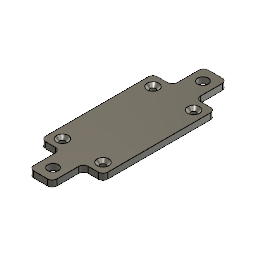
Hoverboard Final v3 (Autodesk Fusion 360 archive; units mm, degrees)
design "RPI PSU Bracket"
Autodesk Fusion 360 part; units mm, degrees
sketch "Sketch1" plane through (0, 0, 0) normal (0, 1, 0) x (1, 0, 0)
  line L0 (13, 29) -> (-13, 29) construction
  line L1 (-13, 29) -> (-13, -29) construction
  line L2 (-13, -29) -> (13, -29) construction
  line L3 (13, -29) -> (13, 29) construction
  line L4 (13, 29) -> (-13, -29) construction
  line L5 (-13, 29) -> (13, -29) construction
  line L6 (0, 0) -> (0, 16.0365) construction
  line L7 (0, 0) -> (-11.1519, 0) construction
  line L8 (20, 36) -> (-20, 36)
  line L9 (-20, 36) -> (-20, -36)
  line L10 (-20, -36) -> (20, -36)
  line L11 (20, -36) -> (20, 36)
  line L12 (20, 36) -> (-20, -36) construction
  line L13 (-20, 36) -> (20, -36) construction
  circle A0 centre (13, 29) radius 1.75
  circle A1 centre (-13, 29) radius 1.75
  circle A2 centre (13, -29) radius 1.75
  circle A3 centre (-13, -29) radius 1.75
  line L14 (7.5, 36) -> (-7.5, 36)
  line L15 (-7.5, 36) -> (-7.5, 56)
  line L16 (-7.5, 56) -> (7.5, 56)
  line L17 (7.5, 56) -> (7.5, 36)
  line L18 (7.5, 36) -> (-7.5, 56) construction
  line L19 (-7.5, 36) -> (7.5, 56) construction
  circle A4 centre (0, 48) radius 3.4
  line L20 (7.5, -56) -> (7.5, -36)
  line L21 (-7.5, -56) -> (7.5, -56)
  line L22 (-7.5, -36) -> (-7.5, -56)
  circle A5 centre (0, -48) radius 3.4
  line L23 (7.5, -36) -> (-7.5, -36)
  point P0 (0, 46)
  dimension "d1" = 3.5
  dimension "d2" = 58
  dimension "d3" = 26
  dimension "d4" = 7
  dimension "d5" = 7
  dimension "d6" = 15
  dimension "d7" = 20
  dimension "d8" = 6.8
  dimension "d9" = 12
  constraint perpendicular L0 L1
  constraint parallel L0 L2
  constraint parallel L1 L3
  constraint horizontal L0
  constraint coincident L4 L6.start
  constraint coincident L5 L6.start
  constraint coincident L6.start L7.start
  constraint vertical L6
  constraint perpendicular L1 L7
  constraint perpendicular L8 L9
  constraint parallel L8 L10
  constraint parallel L9 L11
  constraint horizontal L8
  constraint coincident L12 L6.start
  constraint coincident L13 L6.start
  constraint coincident L0.start L3.end
  constraint symmetric L6 A0 A1
  constraint symmetric L7 A0 A2
  constraint symmetric L7 A1 A3
  constraint perpendicular L14 L15
  constraint parallel L14 L16
  constraint parallel L15 L17
  constraint horizontal L14
  constraint coincident L18 P0
  constraint coincident L19 P0
  constraint coincident L6 P0
  constraint coincident L8 L14.start
  constraint coincident L6 A4.centre
  constraint symmetric L7 L14.start L20.end
  constraint symmetric L7 L14.end L22.start
  constraint symmetric L7 L15.end L21.start
  constraint symmetric L7 L16.end L20.start
  constraint symmetric L7 A4 A5
  measures "d1" diameter of A0
  measures "d2" distance of L0.start L2.end
  measures "d3" distance of L0.start L0.end
  measures "d4" distance of L0 L8
  measures "d5" distance of L3 L11
  measures "d6" distance of L15.end L16.end
  measures "d7" distance of L14.start L16.end
  measures "d8" diameter of A4
  measures "d9" distance of L8 A4.centre
extrude "Extrude1" add sketch "Sketch1" along normal blind 4
fillet "Fillet1" radius 3 12 edges at (7.5, 2, 36) (20, 2, 36) (7.5, 2, 56) (-7.5, 2, 56) (-20, 2, 36) (-7.5, 2, 36) (20, 2, -36) (7.5, 2, -36) (7.5, 2, -56) (-7.5, 2, -56) (-20, 2, -36) (-7.5, 2, -36)
chamfer "Chamfer1" distance 2 angle 45 4 edges at (-14.6316, 4, -29.6328) (11.3684, 4, -29.6328) (11.3684, 4, 28.3672) (-14.6316, 4, 28.3672)

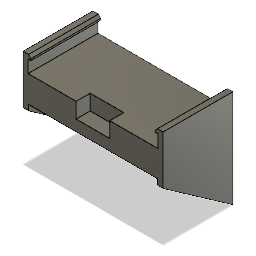
design "Sonar Bracket"
Autodesk Fusion 360 part; units mm, degrees
sketch "Sketch1" plane through (0, 0, 0) normal (0, 1, 0) x (1, 0, 0)
  line L0 (25, -12.5) -> (-25, -12.5)
  line L1 (-25, -12.5) -> (-25, 12.5)
  line L2 (-25, 12.5) -> (25, 12.5)
  line L3 (25, 12.5) -> (25, -12.5)
  line L4 (25, -12.5) -> (-25, 12.5) construction
  line L5 (-25, -12.5) -> (25, 12.5) construction
  dimension "d1" = 25
  dimension "d2" = 50
  constraint perpendicular L0 L1
  constraint parallel L0 L2
  constraint parallel L1 L3
  constraint horizontal L0
  constraint coincident L4 origin
  constraint coincident L5 origin
  measures "d1" distance of L0.end L1.end
  measures "d2" distance of L1.end L2.end
extrude "Extrude1" add sketch "Sketch1" along normal blind 35
sketch "Sketch2" plane through (0, 0, 12.5) normal (0, 0, 1) x (1, 0, 0)
  line L0 (-25, 0) -> (25, 0)
  line L1 (25, 0) -> (25, 35)
  line L2 (25, 35) -> (-25, 35)
  line L3 (-25, 35) -> (-25, 0)
  line L4 (0, 0) -> (0, 11) construction
  line L5 (23, 35) -> (22.15, 34.1)
  line L6 (22.15, 34.1) -> (22.15, 33.5)
  line L7 (22.15, 33.5) -> (23.15, 33.5)
  line L8 (23.15, 33.5) -> (23.15, 29)
  line L9 (23.15, 29) -> (0, 29)
  line L10 (23, 35) -> (0, 35)
  line L11 (-25, 35) -> (25, 35)
  line L12 (-23.15, 33.5) -> (-23.15, 29)
  line L13 (-25, 0) -> (-25, 35)
  line L14 (-23, 35) -> (0, 35)
  line L15 (-22.15, 33.5) -> (-23.15, 33.5)
  line L16 (-22.15, 34.1) -> (-22.15, 33.5)
  line L17 (-23.15, 29) -> (0, 29)
  line L18 (-23, 35) -> (-22.15, 34.1)
  dimension "d5" = 46.3
  dimension "d6" = 1
  dimension "d7" = 1.5
  dimension "d8" = 0.6
  dimension "d9" = 2
  dimension "d10" = 4.5
  constraint coincident L4.start origin
  constraint perpendicular L0 L4
  constraint coincident L2 L5.start
  constraint perpendicular L2 L6
  constraint perpendicular L6 L7
  constraint perpendicular L7 L8
  constraint perpendicular L6 L9
  constraint midpoint L2 L10.end
  constraint symmetric L0.end L4 L0.start
  constraint symmetric L1.end L4 L2.end
  constraint symmetric L2.end L4 L1.end
  constraint symmetric L4 L5.start L14.start
  constraint symmetric L4 L5.end L16.start
  constraint symmetric L4 L6.end L15.start
  constraint symmetric L4 L7.end L12.start
  constraint symmetric L4 L8.end L12.end
  constraint symmetric L4 L9.end L17.end
  constraint symmetric L4 L10.end L14.end
  measures "d5" distance of L8 L12
  measures "d6" distance of L6.end L7.end
  measures "d7" distance of L7.end L10
  measures "d8" distance of L5.end L6.end
  measures "d9" distance of L5.start L1.end
  measures "d10" distance of L7.end L8.end
extrude "Extrude2" cut sketch "Sketch2" against normal through all contours L2 L5 L6 L7 L8 L9 L10 L11 L12 L14 L15 L16 L17 L18
sketch "Sketch3" plane through (0, 0, 12.5) normal (0, 0, 1) x (1, 0, 0)
  line L0 (23, 35) -> (22.15, 34.1)
  line L1 (22.15, 34.1) -> (22.15, 33.5)
  line L2 (22.15, 33.5) -> (23.15, 33.5)
  line L3 (23.15, 33.5) -> (23.15, 29)
  line L4 (23.15, 29) -> (-23.15, 29)
  line L5 (-23.15, 29) -> (-23.15, 33.5)
  line L6 (-23.15, 33.5) -> (-22.15, 33.5)
  line L7 (-22.15, 33.5) -> (-22.15, 34.1)
  line L8 (-22.15, 34.1) -> (-23, 35)
  line L9 (-23, 35) -> (-25, 35)
  line L10 (-25, 35) -> (-25, 0)
  line L11 (-25, 0) -> (25, 0)
  line L12 (25, 0) -> (25, 35)
  line L13 (25, 35) -> (23, 35)
  line L14 (6, 23.5) -> (-6, 23.5)
  line L15 (-6, 23.5) -> (-6, 34.5)
  line L16 (-6, 34.5) -> (6, 34.5)
  line L17 (6, 34.5) -> (6, 23.5)
  line L18 (6, 23.5) -> (-6, 34.5) construction
  line L19 (-6, 23.5) -> (6, 34.5) construction
  point P0 (0, 29)
  dimension "d12" = 12
  dimension "d13" = 11
  constraint perpendicular L14 L15
  constraint parallel L14 L16
  constraint parallel L15 L17
  constraint horizontal L14
  constraint coincident L18 P0
  constraint coincident L19 P0
  constraint midpoint L4 P0
  measures "d12" distance of L14.start L14.end
  measures "d13" distance of L14.start L16.end
extrude "Extrude3" cut sketch "Sketch3" against normal blind 5 contours L4 L14 L15 L17
sketch "Sketch4" plane through (25, 0, 0) normal (1, 0, 0) x (0, 0, -1)
  line L0 (-12.5, 0) -> (12.5, 0)
  line L1 (12.5, 0) -> (12.5, 35)
  line L2 (12.5, 35) -> (-12.5, 35)
  line L3 (-12.5, 35) -> (-12.5, 0)
  line L4 (-12.5, 17.5) -> (12.5, 0)
  line L5 (12.5, 0) -> (-12.5, 0)
  line L6 (-12.5, 0) -> (-12.5, 17.5)
  constraint midpoint L3 L4.start
  constraint coincident L0.end L1.start
  constraint coincident L0.start L3.end
extrude "Extrude4" cut sketch "Sketch4" against normal through all contours L0 L3 L4 L5 L6
sketch "Sketch5" plane through (0, 0, 12.5) normal (0, 0, 1) x (1, 0, 0)
  line L0 (-25, 17.5) -> (25, 17.5)
  line L1 (25, 17.5) -> (25, 35)
  line L2 (25, 35) -> (23, 35)
  line L3 (23, 35) -> (22.15, 34.1)
  line L4 (22.15, 34.1) -> (22.15, 33.5)
  line L5 (22.15, 33.5) -> (23.15, 33.5)
  line L6 (23.15, 33.5) -> (23.15, 29)
  line L7 (23.15, 29) -> (6, 29)
  line L8 (6, 29) -> (6, 23.5)
  line L9 (6, 23.5) -> (-6, 23.5)
  line L10 (-6, 23.5) -> (-6, 29)
  line L11 (-6, 29) -> (-23.15, 29)
  line L12 (-23.15, 29) -> (-23.15, 33.5)
  line L13 (-23.15, 33.5) -> (-22.15, 33.5)
  line L14 (-22.15, 33.5) -> (-22.15, 34.1)
  line L15 (-22.15, 34.1) -> (-23, 35)
  line L16 (-23, 35) -> (-25, 35)
  line L17 (-25, 35) -> (-25, 17.5)
  line L18 (23, 19.5) -> (-23, 19.5)
  line L19 (-23, 19.5) -> (-23, 0)
  line L20 (-23, 0) -> (23, 0)
  line L21 (23, 0) -> (23, 19.5)
  line L22 (23, 19.5) -> (-23, 0) construction
  line L23 (-23, 19.5) -> (23, 0) construction
  line L24 (-25, 0) -> (25, 0)
  line L25 (25, 17.5) -> (25, 0)
  line L26 (-25, 0) -> (-25, 17.5)
  point P0 (0, 9.75)
  dimension "d17" = 2
  dimension "d18" = 2
  dimension "d19" = 2
  constraint perpendicular L18 L19
  constraint parallel L18 L20
  constraint parallel L19 L21
  constraint horizontal L18
  constraint coincident L22 P0
  constraint coincident L23 P0
  constraint collinear L20 L24
  measures "d17" distance of L0 L18
  measures "d18" distance of L21 L25
  measures "d19" distance of L19 L26
extrude "Extrude5" cut sketch "Sketch5" against normal blind 21 contours L0 L18 L19 L21 | L0 L19 L20 L21 L24
sketch "Sketch6" plane through (0, 0, -8.5) normal (0, 0, 1) x (1, 0, 0)
  line L0 (-23, 2.8) -> (23, 2.8)
  line L1 (23, 2.8) -> (23, 19.5)
  line L2 (23, 19.5) -> (-23, 19.5)
  line L3 (-23, 19.5) -> (-23, 2.8)
  circle A0 centre (0, 9.5) radius 3.25
  line L4 (0, 0) -> (0, 14) construction
  dimension "d22" = 6.5
  dimension "d23" = 9.5
  constraint coincident L4.start origin
  constraint vertical L4
  constraint coincident A0.centre L4
  measures "d22" diameter of A0
  measures "d23" distance of L4.start A0.centre
extrude "Extrude6" cut sketch "Sketch6" against normal through all contours A0

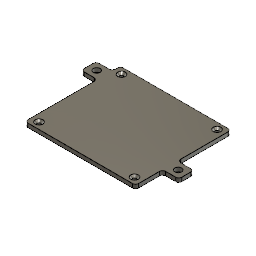
design "Power PCB Bracket"
Autodesk Fusion 360 part; units mm, degrees
sketch "Sketch1" plane through (0, 0, 0) normal (0, 1, 0) x (1, 0, 0)
  line L0 (47.35, 40.9) -> (-47.35, 40.9) construction
  line L1 (-47.35, 40.9) -> (-47.35, -40.9) construction
  line L2 (-47.35, -40.9) -> (47.35, -40.9) construction
  line L3 (47.35, -40.9) -> (47.35, 40.9) construction
  line L4 (47.35, 40.9) -> (-47.35, -40.9) construction
  line L5 (-47.35, 40.9) -> (47.35, -40.9) construction
  line L6 (54.9177, 47.4368) -> (-54.9177, 47.4368)
  line L7 (-54.9177, 47.4368) -> (-54.9177, -47.4368)
  line L8 (-54.9177, -47.4368) -> (54.9177, -47.4368)
  line L9 (54.9177, -47.4368) -> (54.9177, 47.4368)
  line L10 (54.9177, 47.4368) -> (-54.9177, -47.4368) construction
  line L11 (-54.9177, 47.4368) -> (54.9177, -47.4368) construction
  circle A0 centre (47.35, 40.9) radius 1.75
  line L12 (0, 0) -> (0, 35) construction
  line L13 (0, 0) -> (-41.0628, 0) construction
  circle A1 centre (-47.35, 40.9) radius 1.75
  circle A2 centre (47.35, -40.9) radius 1.75
  circle A3 centre (-47.35, -40.9) radius 1.75
  line L14 (-54.9177, 39.4) -> (-70.9177, 39.4)
  line L15 (-70.9177, 39.4) -> (-70.9177, 24.4)
  line L16 (-70.9177, 24.4) -> (-54.9177, 24.4)
  line L17 (-54.9177, 24.4) -> (-54.9177, 39.4)
  line L18 (54.9177, -5.6) -> (70.9177, -5.6)
  line L19 (70.9177, -5.6) -> (70.9177, -20.6)
  line L20 (70.9177, -20.6) -> (54.9177, -20.6)
  line L21 (54.9177, -20.6) -> (54.9177, -5.6)
  line L22 (81.8257, 31.9) -> (62.2169, 31.9) construction
  line L23 (80.3912, -13.1) -> (59.348, -13.1) construction
  circle A4 centre (-62.9177, 31.9) radius 3.4
  circle A5 centre (62.9177, -13.1) radius 3.4
  dimension "d1" = 3.5
  dimension "d2" = 81.8
  dimension "d3" = 94.7
  dimension "d4" = 10
  dimension "d5" = 16
  dimension "d6" = 15
  dimension "d7" = 15
  dimension "d9" = 16
  dimension "d10" = 45
  dimension "d11" = 9
  dimension "d12" = 6.8
  dimension "d13" = 6.8
  dimension "d14" = 8
  dimension "d15" = 8
  constraint perpendicular L0 L1
  constraint parallel L0 L2
  constraint parallel L1 L3
  constraint horizontal L0
  constraint coincident L4 L12.start
  constraint coincident L5 L12.start
  constraint coincident L12.start L13.start
  constraint perpendicular L6 L7
  constraint parallel L6 L8
  constraint parallel L7 L9
  constraint horizontal L6
  constraint coincident L10 L12.start
  constraint coincident L11 L12.start
  constraint collinear L4 L10
  constraint coincident L0.start L3.end
  constraint vertical L12
  constraint horizontal L13
  constraint symmetric A0 L12 A1
  constraint symmetric A0 L13 A2
  constraint symmetric L13 A1 A3
  constraint horizontal L14
  constraint vertical L15
  constraint horizontal L16
  constraint vertical L17
  constraint coincident L7 L14.start
  constraint horizontal L18
  constraint vertical L19
  constraint horizontal L20
  constraint vertical L21
  constraint coincident L9 L18.start
  constraint perpendicular L12 L22
  constraint symmetric L14 L16 L22
  constraint symmetric L18 L20 L23
  constraint coincident L23 A5.centre
  constraint coincident L22 A4.centre
  measures "d1" diameter of A0
  measures "d2" distance of L0.start L2.end
  measures "d3" distance of L0.start L0.end
  measures "d4" distance of L6.start L0.start
  measures "d5" distance of L14.start L14.end
  measures "d6" distance of L14.end L15.end
  measures "d7" distance of L18.end L19.end
  measures "d9" distance of L18.start L18.end
  measures "d10" distance of L22 L23
  measures "d11" distance of L0.end L22
  measures "d12" diameter of A5
  measures "d13" diameter of A4
  measures "d14" distance of L7 A4.centre
  measures "d15" distance of L21 A5.centre
extrude "Extrude1" add sketch "Sketch1" along normal blind 4
fillet "Fillet1" radius 3 12 edges at (-70.9177, 2, -24.4) (-70.9177, 2, -39.4) (-54.9177, 2, -39.4) (-54.9177, 2, -47.4368) (-54.9177, 2, 47.4368) (-54.9177, 2, -24.4) (54.9177, 2, 47.4368) (54.9177, 2, 20.6) (70.9177, 2, 20.6) (70.9177, 2, 5.6) (54.9177, 2, 5.6) (54.9177, 2, -47.4368)
chamfer "Chamfer1" distance 2 angle 45 4 edges at (45.7184, 4, 40.2672) (-48.9816, 4, 40.2672) (-48.9816, 4, -41.5328) (45.7184, 4, -41.5328)

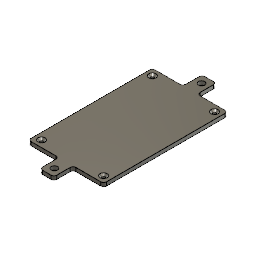
design "PSU Bracket"
Autodesk Fusion 360 part; units mm, degrees
sketch "Sketch1" plane through (0, 0, 0) normal (0, 1, 0) x (1, 0, 0)
  line L0 (32.5, 58) -> (-32.5, 58) construction
  line L1 (-32.5, 58) -> (-32.5, -58) construction
  line L2 (-32.5, -58) -> (32.5, -58) construction
  line L3 (32.5, -58) -> (32.5, 58) construction
  line L4 (32.5, 58) -> (-32.5, -58) construction
  line L5 (-32.5, 58) -> (32.5, -58) construction
  circle A0 centre (32.5, 58) radius 1.75
  line L6 (0, 0) -> (0, 14) construction
  line L7 (0, 0) -> (-15, 0) construction
  circle A1 centre (-32.5, 58) radius 1.75
  circle A2 centre (32.5, -58) radius 1.75
  circle A3 centre (-32.5, -58) radius 1.75
  line L8 (39.5, 65) -> (-39.5, 65)
  line L9 (-39.5, 65) -> (-39.5, -65)
  line L10 (-39.5, -65) -> (39.5, -65)
  line L11 (39.5, -65) -> (39.5, 65)
  line L12 (39.5, 65) -> (-39.5, -65) construction
  line L13 (-39.5, 65) -> (39.5, -65) construction
  line L14 (7.5, 85) -> (-7.5, 85)
  line L15 (-7.5, 85) -> (-7.5, 65)
  line L16 (-7.5, 65) -> (7.5, 65)
  line L17 (7.5, 65) -> (7.5, 85)
  line L18 (7.5, 85) -> (-7.5, 65) construction
  line L19 (-7.5, 85) -> (7.5, 65) construction
  circle A4 centre (0, 77) radius 3.25
  line L20 (-7.5, -85) -> (-7.5, -65)
  line L21 (7.5, -85) -> (-7.5, -85)
  line L22 (-7.5, -85) -> (7.5, -65) construction
  circle A5 centre (0, -77) radius 3.25
  line L23 (-7.5, -65) -> (7.5, -65)
  line L24 (7.5, -65) -> (7.5, -85)
  line L25 (7.5, -85) -> (-7.5, -65) construction
  point P0 (0, 75)
  point P1 (0, -75)
  dimension "d1" = 116
  dimension "d2" = 65
  dimension "d3" = 3.5
  dimension "d4" = 7
  dimension "d5" = 7
  dimension "d6" = 20
  dimension "d7" = 15
  dimension "d8" = 6.5
  dimension "d9" = 12
  constraint perpendicular L0 L1
  constraint parallel L0 L2
  constraint parallel L1 L3
  constraint horizontal L0
  constraint coincident L4 L6.start
  constraint coincident L5 L6.start
  constraint coincident L6.start L7.start
  constraint coincident L0.start L3.end
  constraint vertical L6
  constraint perpendicular L6 L7
  constraint symmetric A0 L6 A1
  constraint symmetric A0 L7 A2
  constraint symmetric L7 A1 A3
  constraint perpendicular L8 L9
  constraint parallel L8 L10
  constraint parallel L9 L11
  constraint horizontal L8
  constraint coincident L12 L6.start
  constraint coincident L13 L6.start
  constraint perpendicular L14 L15
  constraint parallel L14 L16
  constraint parallel L15 L17
  constraint horizontal L14
  constraint coincident L18 P0
  constraint coincident L19 P0
  constraint collinear L8 L16
  constraint coincident L6 P0
  constraint coincident L6 A4.centre
  constraint symmetric L7 L14.start L21.start
  constraint symmetric L7 L14.end L20.start
  constraint symmetric L7 L15.end L20.end
  constraint symmetric L7 L16.end L22.end
  constraint symmetric L7 P0 P1
  constraint symmetric L7 A4 A5
  measures "d1" distance of L0.start L2.end
  measures "d2" distance of L0.start L0.end
  measures "d3" diameter of A0
  measures "d4" distance of L0.start L8
  measures "d5" distance of L0.start L11
  measures "d6" distance of L14 L16
  measures "d7" distance of L15 L17
  measures "d8" diameter of A4
  measures "d9" distance of L8 A4.centre
extrude "Extrude1" add sketch "Sketch1" along normal blind 4
fillet "Fillet1" radius 3 12 edges at (-39.5, 2, 65) (-7.5, 2, 85) (7.5, 2, 85) (7.5, 2, 65) (39.5, 2, 65) (39.5, 2, -65) (7.5, 2, -65) (7.5, 2, -85) (-7.5, 2, -85) (-39.5, 2, -65) (-7.5, 2, -65) (-7.5, 2, 65)
chamfer "Chamfer2" distance 2 angle 45 4 edges at (-34.1316, 4, 57.3672) (30.8684, 4, 57.3672) (30.8684, 4, -58.6328) (-34.1316, 4, -58.6328)

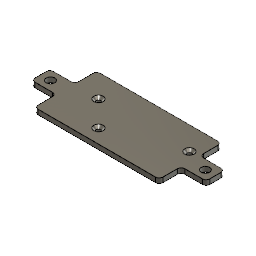
design "Sonar PCB Bracket"
Autodesk Fusion 360 part; units mm, degrees
sketch "Sketch1" plane through (0, 0, 0) normal (0, 1, 0) x (1, 0, 0)
  line L0 (50, 25) -> (-50, 25)
  line L1 (-50, 25) -> (-50, -25)
  line L2 (-50, -25) -> (50, -25)
  line L3 (50, -25) -> (50, 25)
  line L4 (50, 25) -> (-50, -25) construction
  line L5 (-50, 25) -> (50, -25) construction
  line L6 (0, 0) -> (0, 15) construction
  line L7 (0, 0) -> (-17.4892, 0) construction
  circle A0 centre (42.83, 6.35) radius 1.75
  circle A1 centre (-30, 6.35) radius 1.75
  circle A2 centre (-9.85, -13.8) radius 1.75
  line L8 (70, 7.5) -> (50, 7.5)
  line L9 (50, 7.5) -> (50, -7.5)
  line L10 (50, -7.5) -> (70, -7.5)
  line L11 (70, -7.5) -> (70, 7.5)
  line L12 (70, 7.5) -> (50, -7.5) construction
  line L13 (50, 7.5) -> (70, -7.5) construction
  line L14 (-70, 7.5) -> (-50, 7.5)
  line L15 (-70, -7.5) -> (-70, 7.5)
  line L16 (-50, -7.5) -> (-70, -7.5)
  circle A3 centre (62, 0) radius 3.4
  circle A4 centre (-62, 0) radius 3.4
  line L17 (42.83, 6.35) -> (-30, 6.35) construction
  point P0 (60, 0)
  dimension "d1" = 3.5
  dimension "d2" = 3.5
  dimension "d3" = 3.5
  dimension "d4" = 6.8
  dimension "d5" = 15
  dimension "d6" = 20
  dimension "d7" = 12
  dimension "d8" = 100
  dimension "d9" = 50
  dimension "d10" = 72.83
  dimension "d11" = 20.15
  dimension "d12" = 20.15
  dimension "d13" = 20
  dimension "d14" = 18.65
  constraint perpendicular L0 L1
  constraint parallel L0 L2
  constraint parallel L1 L3
  constraint horizontal L0
  constraint coincident L4 L6.start
  constraint coincident L5 L6.start
  constraint coincident L6.start L7.start
  constraint vertical L6
  constraint perpendicular L6 L7
  constraint perpendicular L8 L9
  constraint parallel L8 L10
  constraint parallel L9 L11
  constraint horizontal L8
  constraint coincident L12 P0
  constraint coincident L13 P0
  constraint coincident L7 P0
  constraint collinear L3 L9
  constraint symmetric L6 L8.start L14.start
  constraint symmetric L6 L8.end L14.end
  constraint symmetric L6 L9.end L16.start
  constraint symmetric L6 L10.end L15.start
  constraint coincident L7 A3.centre
  constraint symmetric L6 A3 A4
  constraint coincident A0.centre L17.start
  constraint coincident A1.centre L17.end
  constraint horizontal L17
  measures "d1" diameter of A2
  measures "d2" diameter of A1
  measures "d3" diameter of A0
  measures "d4" diameter of A3
  measures "d5" distance of L8.start L10.end
  measures "d6" distance of L8.start L8.end
  measures "d7" distance of L3 A3.centre
  measures "d8" distance of L0.start L0.end
  measures "d9" distance of L0.start L2.end
  measures "d10" horizontal distance of A0.centre A1.centre
  measures "d11" vertical distance of A1.centre A2.centre
  measures "d12" horizontal distance of A1.centre A2.centre
  measures "d13" distance of L1 A1.centre
  measures "d14" distance of L0 A1.centre
extrude "Extrude1" add sketch "Sketch1" along normal blind 4
fillet "Fillet1" radius 3 12 edges at (50, 2, 7.5) (50, 2, 25) (70, 2, 7.5) (70, 2, -7.5) (50, 2, -7.5) (50, 2, -25) (-50, 2, -25) (-50, 2, -7.5) (-70, 2, -7.5) (-70, 2, 7.5) (-50, 2, 7.5) (-50, 2, 25)
chamfer "Chamfer1" distance 2 angle 45 3 edges at (41.1984, 4, -6.9828) (-11.4816, 4, 13.1672) (-31.6316, 4, -6.9828)

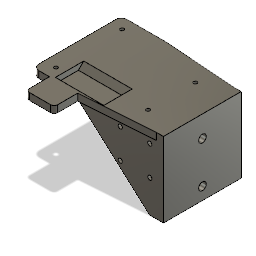
design "RPLIDAR Bracket"
Autodesk Fusion 360 part; units mm, degrees
sketch "Sketch1" plane through (0, 0, 0) normal (0, 1, 0) x (1, 0, 0)
  line L0 (0, 0) -> (-5, 0) construction
  line L1 (-5, 0) -> (-33.0162, 0) construction
  line L2 (0, 0) -> (0, 35) construction
  circle A0 centre (-28, 28) radius 1.5
  circle A1 centre (42, 20) radius 1.5
  circle A2 centre (-28, -28) radius 1.5
  circle A3 centre (42, -20) radius 1.5
  line L3 (-38, 0) -> (-38, 37.5)
  line L4 (-38, 37.5) -> (0, 37.5)
  line L5 (0, 37.5) -> (62, 33)
  line L6 (62, 33) -> (62, 0)
  line L7 (62, -33) -> (62, 0)
  line L8 (0, -37.5) -> (62, -33)
  line L9 (-38, -37.5) -> (0, -37.5)
  line L10 (-38, 0) -> (-38, -37.5)
  dimension "d1" = 3
  dimension "d2" = 3
  dimension "d3" = 40
  dimension "d4" = 56
  dimension "d5" = 70
  dimension "d6" = 42
  dimension "d7" = 75
  dimension "d8" = 100
  dimension "d9" = 10
  dimension "d10" = 33
  constraint coincident L0.start L2.start
  constraint horizontal L0
  constraint parallel L0 L1
  constraint perpendicular L0 L2
  constraint symmetric L1 A0 A2
  constraint symmetric L1 A1 A3
  constraint perpendicular L2 L4
  constraint parallel L2 L6
  constraint symmetric L1 L3.start L10.start
  constraint symmetric L1 L3.end L9.start
  constraint symmetric L1 L4.end L8.start
  constraint symmetric L1 L5.end L7.start
  constraint symmetric L1 L6.end L7.end
  constraint vertical L3
  constraint coincident L2 L4.end
  constraint coincident L6.end L7.end
  constraint coincident L3.start L10.start
  measures "d1" diameter of A0
  measures "d2" diameter of A1
  measures "d3" distance of A1.centre A3.centre
  measures "d4" distance of A0.centre A2.centre
  measures "d5" horizontal distance of A0.centre A1.centre
  measures "d6" horizontal distance of L0.start A1.centre
  measures "d7" distance of L3.end L9.start
  measures "d8" distance of L3 L6
  measures "d9" distance of A0.centre L3
  measures "d10" distance of L5.end L6.end
  measures "d20" angle of L4.end
extrude "Extrude1" add sketch "Sketch1" along normal blind 6
ref_plane "WorkPlane1" through (0, 0, 27) normal (0, 0, 1) x (1, 0, 0)
sketch "Sketch3" plane through (0, 0, 27) normal (0, 0, 1) x (1, 0, 0)
  line L0 (-8, 0) -> (62, 0)
  line L1 (62, -57.6259) -> (56, -57.6259)
  line L2 (56, -57.6259) -> (-8, 0)
  line L3 (62, 0) -> (62, -57.6259)
  line L4 (54.1896, -11.7055) -> (54.187, -11.7094)
  point P0 (5, 0)
  dimension "d19" = 6
  dimension "d20" = 42
  dimension "d21" = 70
  constraint vertical L3
  constraint perpendicular L0 L3
  constraint coincident L0.end L4
  constraint perpendicular L1 L3
  constraint coincident P0 L0
  constraint coincident origin L0
  measures "d19" distance of L1.end L1.start
  measures "d20" angle of L0 L2
  measures "d21" distance of L0.start L0.end
extrude "Extrude3" add sketch "Sketch3" along normal blind 6
mirror "Mirror1" about plane through (0, 0, 0) normal (0, 0, 1) of "Extrude3"
sketch "Sketch4" plane through (62, 0, 0) normal (1, 0, 0) x (0, 0, -1)
  line L0 (-27, 0) -> (27, 0)
  line L1 (27, 0) -> (27, -57.6259)
  line L2 (27, -57.6259) -> (33, -57.6259)
  line L3 (33, -57.6259) -> (33, 0)
  line L4 (-33, 0) -> (-33, -57.6259)
  line L5 (-33, -57.6259) -> (-27, -57.6259)
  line L6 (-27, -57.6259) -> (-27, 0)
  line L7 (-33, 6) -> (33, 6)
  line L8 (33, 6) -> (33, -57.6259)
  line L9 (33, -57.6259) -> (-33, -57.6259)
  line L10 (-33, -57.6259) -> (-33, 6)
  circle A0 centre (0, -12) radius 3.25
  circle A1 centre (0, -47) radius 3.25
  line L11 (33, 0) -> (33, 6)
  line L12 (33, 6) -> (-33, 6)
  line L13 (-33, 6) -> (-33, 0)
  dimension "d27" = 6.5
  dimension "d28" = 6.5
  dimension "d29" = 35
  dimension "d30" = 12
  constraint horizontal L7
  constraint vertical L8
  constraint horizontal L9
  constraint vertical L10
  constraint coincident L2.end L3.start
  measures "d27" diameter of A1
  measures "d28" diameter of A0
  measures "d29" distance of A0.centre A1.centre
  measures "d30" distance of L0 A0.centre
extrude "Extrude4" add sketch "Sketch4" along normal blind 6
fillet "Fillet1" radius 5 2 edges at (-38, 3, 37.5) (-38, 3, -37.5)
sketch "Sketch5" plane through (0, 6, 0) normal (0, 1, 0) x (-1, 0, 0)
  arc A0 (33, -37.5) -> (38, -32.5) centre (33, -32.5) ccw
  line L0 (38, -32.5) -> (38, 32.5)
  arc A1 (38, 32.5) -> (33, 37.5) centre (33, 32.5) ccw
  line L1 (33, 37.5) -> (0, 37.5)
  line L2 (0, 37.5) -> (-62, 33)
  line L3 (-62, 33) -> (-68, 33)
  line L4 (0, -37.5) -> (33, -37.5)
  circle A2 centre (28, 28) radius 1.5
  circle A3 centre (-42, 20) radius 1.5
  circle A4 centre (28, -28) radius 1.5
  line L5 (24, 37.5) -> (24, 57.5)
  line L6 (24, 57.5) -> (0, 57.5)
  line L7 (0, 57.5) -> (0, 37.5)
  line L8 (0, 37.5) -> (24, 37.5)
  dimension "d32" = 20
  dimension "d33" = 24
  constraint coincident L1 L5.start
  constraint perpendicular L1 L5
  constraint coincident L1.end L2.start
  constraint perpendicular L1 L7
  constraint horizontal L6
  measures "d32" distance of L5.start L5.end
  measures "d33" distance of L5.end L6.end
extrude "Extrude5" add sketch "Sketch5" against normal blind 6 contours L1 L5 L6 L7 L8
fillet "Fillet2" radius 3 2 edges at (-24, 3, 57.5) (0, 3, 57.5)
sketch "Sketch6" plane through (0, 6, 0) normal (0, 1, 0) x (-1, 0, 0)
  arc A0 (3, 57.5) -> (0, 54.5) centre (3, 54.5) ccw
  line L0 (0, 54.5) -> (0, 37.5)
  line L1 (0, 37.5) -> (-62, 33)
  line L2 (-62, 33) -> (-68, 33)
  line L3 (-68, 33) -> (-68, -33)
  line L4 (-68, -33) -> (-62, -33)
  line L5 (-62, -33) -> (0, -37.5)
  line L6 (0, -37.5) -> (33, -37.5)
  arc A1 (33, -37.5) -> (38, -32.5) centre (33, -32.5) ccw
  line L7 (38, -32.5) -> (38, 32.5)
  arc A2 (38, 32.5) -> (33, 37.5) centre (33, 32.5) ccw
  line L8 (33, 37.5) -> (24, 37.5)
  line L9 (24, 37.5) -> (24, 54.5)
  arc A3 (24, 54.5) -> (21, 57.5) centre (21, 54.5) ccw
  line L10 (21, 57.5) -> (3, 57.5)
  circle A4 centre (28, 28) radius 1.5
  circle A5 centre (-42, 20) radius 1.5
  circle A6 centre (-42, -20) radius 1.5
  circle A7 centre (28, -28) radius 1.5
  line L11 (21, 16) -> (-20, 16)
  line L12 (-20, 16) -> (-20, 30.9726)
  line L13 (-20, 30.9726) -> (21, 30.9726)
  line L14 (21, 30.9726) -> (21, 16)
  constraint horizontal L11
  constraint vertical L12
  constraint horizontal L13
  constraint vertical L14
extrude "Extrude6" cut sketch "Sketch6" against normal blind 4.5 contours L11 L12 L13 L14
chamfer "Chamfer1" distance 4.5 angle 45 2 edges at (-0.5, 6, 30.9726) (-0.5, 6, 16)
sketch "Sketch7" plane through (0, 0, 33) normal (0, 0, 1) x (1, 0, 0)
  line L0 (62, 0) -> (-8, 0)
  line L1 (-8, 0) -> (56, -57.6259) construction
  line L2 (56, -57.6259) -> (68, -57.6259)
  line L3 (68, -57.6259) -> (68, 6) construction
  line L4 (68, 6) -> (62, 6)
  line L5 (62, 6) -> (62, 0)
  line L6 (56.4712, -5.0375) -> (31.4712, -5.0375) construction
  line L7 (31.4712, -5.0375) -> (31.4712, -30.0375) construction
  line L8 (31.4712, -30.0375) -> (56.4712, -30.0375) construction
  line L9 (56.4712, -30.0375) -> (56.4712, -5.0375) construction
  line L10 (56.4712, -5.0375) -> (31.4712, -30.0375) construction
  line L11 (31.4712, -5.0375) -> (56.4712, -30.0375) construction
  circle A0 centre (56.4712, -5.0375) radius 1.75
  line L12 (43.9712, -17.5375) -> (43.9712, -12) construction
  line L13 (43.9712, -17.5375) -> (51.6365, -17.5375) construction
  circle A1 centre (31.4712, -5.0375) radius 1.75
  circle A2 centre (31.4712, -30.0375) radius 1.75
  circle A3 centre (56.4712, -30.0375) radius 1.75
  point P0 (43.9712, -17.5375)
  dimension "d43" = 25
  dimension "d44" = 25
  dimension "d45" = 3.5
  constraint perpendicular L6 L7
  constraint parallel L6 L8
  constraint parallel L7 L9
  constraint horizontal L6
  constraint coincident L10 P0
  constraint coincident L11 P0
  constraint coincident L6.start L9.end
  constraint coincident P0 L12.start
  constraint perpendicular L8 L12
  constraint perpendicular L12 L13
  constraint symmetric A0 L12 A1
  constraint symmetric A0 L13 A3
  constraint symmetric L13 A1 A2
  measures "d43" distance of L6.start L8.end
  measures "d44" distance of L6.start L6.end
  measures "d45" diameter of A0
extrude "Extrude7" cut sketch "Sketch7" against normal up to surface (6 mm away)
equation "d5 = 28 mm + 42 mm"

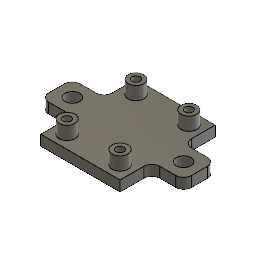
design "Joystick mount"
Autodesk Fusion 360 part; units mm, degrees
sketch "Sketch1" plane through (0, 0, 0) normal (0, 1, 0) x (1, 0, 0)
  line L0 (10, 13) -> (-10, 13) construction
  line L1 (-10, 13) -> (-10, -13) construction
  line L2 (-10, -13) -> (10, -13) construction
  line L3 (10, -13) -> (10, 13) construction
  line L4 (10, 13) -> (-10, -13) construction
  line L5 (-10, 13) -> (10, -13) construction
  circle A0 centre (10, 13) radius 1.5
  line L6 (0, 0) -> (0, 6) construction
  line L7 (0, 0) -> (-6, 0) construction
  line L8 (2.5, 0) -> (20, 0)
  circle A1 centre (10, -13) radius 1.5
  line L9 (0, -20) -> (0, -2.5)
  circle A2 centre (-10, 13) radius 1.5
  circle A3 centre (-10, -13) radius 1.5
  circle A4 centre (-10, -13) radius 3
  circle A5 centre (-10, 13) radius 3
  circle A6 centre (10, -13) radius 3
  circle A7 centre (10, 13) radius 3
  line L10 (15, -18) -> (-15, -18)
  line L11 (-15, -18) -> (-15, 18)
  line L12 (-15, 18) -> (15, 18)
  line L13 (15, 18) -> (15, -18)
  line L14 (15, -18) -> (-15, 18) construction
  line L15 (-15, -18) -> (15, 18) construction
  line L16 (15, -6) -> (27, -6)
  line L17 (27, -6) -> (27, 6)
  line L18 (27, 6) -> (15, 6)
  line L19 (15, 6) -> (15, -6)
  line L20 (15, -6) -> (27, 6) construction
  line L21 (27, -6) -> (15, 6) construction
  circle A8 centre (21, 0) radius 2.75
  circle A9 centre (-21, 0) radius 2.75
  line L22 (-15, -6) -> (-27, -6)
  line L23 (-27, -6) -> (-27, 6)
  line L24 (-27, 6) -> (-15, 6)
  point P0 (21, 0)
  dimension "d1" = 3
  dimension "d2" = 1.5
  dimension "d3" = 26
  dimension "d4" = 20
  dimension "d5" = 5
  dimension "d6" = 5
  dimension "d7" = 12
  dimension "d8" = 12
  dimension "d9" = 5.5
  constraint perpendicular L0 L1
  constraint parallel L0 L2
  constraint parallel L1 L3
  constraint horizontal L0
  constraint coincident L4 L6.start
  constraint coincident L5 L6.start
  constraint coincident L6.start L7.start
  constraint coincident L0.start L3.end
  constraint vertical L6
  constraint perpendicular L6 L7
  constraint symmetric A0 L8 A1
  constraint symmetric A0 L9 A2
  constraint symmetric A1 L9 A3
  constraint concentric A3 A4
  constraint symmetric L8 A4 A5
  constraint symmetric L9 A4 A6
  constraint symmetric L9 A5 A7
  constraint perpendicular L10 L11
  constraint parallel L10 L12
  constraint parallel L11 L13
  constraint horizontal L10
  constraint coincident L14 L6.start
  constraint coincident L15 L6.start
  constraint perpendicular L16 L17
  constraint parallel L16 L18
  constraint parallel L17 L19
  constraint horizontal L16
  constraint coincident L13 L16.start
  constraint coincident L20 P0
  constraint coincident L21 P0
  constraint coincident L8 P0
  constraint coincident P0 A8.centre
  constraint symmetric L9 L16.start L22.start
  constraint symmetric L9 L16.end L22.end
  constraint symmetric L9 L17.end L23.end
  constraint symmetric L9 L18.end L24.end
  constraint symmetric L9 A8 A9
  measures "d1" diameter of A3
  measures "d2" distance of A1 A6
  measures "d3" distance of L2.end L0.start
  measures "d4" distance of L2.end L1.end
  measures "d5" distance of L2.end L10
  measures "d6" distance of L2.end L13
  measures "d7" distance of L17 L19
  measures "d8" distance of L16 L18
  measures "d9" diameter of A8
extrude "Extrude1" add sketch "Sketch1" against normal blind 4 contours A0 | A1 | A2 | A3 | A4 | A5 | A6 | A7 | L10 L11 L12 L13 L19 | L13 L16 L17 L18 L19 | L11 L22 L23 L24
extrude "Extrude2" add sketch "Sketch1" along normal blind 5 contours A4 | A5 | A6 | A7
extrude "Extrude3" cut sketch "Sketch1" against normal blind 3 contours A0 | A1 | A2 | A3
fillet "Fillet1" radius 3 8 edges at (-27, -2, -6) (-27, -2, 6) (27, -2, -6) (27, -2, 6) (15, -2, -6) (15, -2, 6) (-15, -2, 6) (-15, -2, -6)

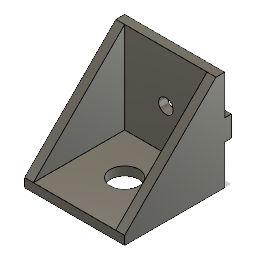
design "Charger Bracket"
Autodesk Fusion 360 part; units mm, degrees
sketch "Sketch1" plane through (0, 0, 0) normal (0, 1, 0) x (1, 0, 0)
  line L0 (22.5, 22.5) -> (-22.5, 22.5)
  line L1 (-22.5, 22.5) -> (-22.5, -22.5)
  line L2 (-22.5, -22.5) -> (22.5, -22.5)
  line L3 (22.5, -22.5) -> (22.5, 22.5)
  line L4 (22.5, 22.5) -> (-22.5, -22.5) construction
  line L5 (-22.5, 22.5) -> (22.5, -22.5) construction
  dimension "d1" = 45
  dimension "d2" = 45
  constraint perpendicular L0 L1
  constraint parallel L0 L2
  constraint parallel L1 L3
  constraint horizontal L0
  constraint coincident L4 origin
  constraint coincident L5 origin
  measures "d1" distance of L0.start L2.end L0.end
  measures "d2" distance of L0.start L0.end
extrude "Extrude1" add sketch "Sketch1" along normal blind 4
sketch "Sketch2" plane through (0, 0, -22.5) normal (0, 0, -1) x (-1, 0, 0)
  line L0 (22.5, 0) -> (-22.5, 0)
  line L1 (-22.5, 0) -> (-22.5, 45)
  line L2 (-22.5, 45) -> (22.5, 45)
  line L3 (22.5, 45) -> (22.5, 0)
  point P0 (-22.5, 0)
  point P1 (22.5, 0)
  dimension "d12" = 45
  constraint horizontal L0
  constraint vertical L1
  constraint horizontal L2
  constraint vertical L3
  constraint coincident L0 P0
  constraint coincident L1 P0
  constraint coincident L3 P1
  measures "d12" distance of P0 L1.end
extrude "Extrude4" add sketch "Sketch2" against normal blind 4
sketch "Sketch3" plane through (-22.5, 0, 0) normal (-1, 0, 0) x (0, 0, 1)
  line L0 (-22.5, 0) -> (22.5, 0)
  line L1 (22.5, 0) -> (22.5, 4)
  line L2 (22.5, 4) -> (-18.5, 4)
  line L3 (-22.5, 45) -> (-22.5, 0)
  line L4 (-18.5, 45) -> (-18.5, 4)
  line L5 (22.5, 4) -> (-18.5, 45)
  line L6 (-18.5, 4) -> (-18.5, 45)
  line L7 (-18.5, 45) -> (-22.5, 45)
  constraint coincident L2.end L4.end
  constraint coincident L1.end L2.start
  constraint coincident L4.start L5.end
extrude "Extrude3" add sketch "Sketch3" against normal blind 4 contours L2 L4 L5 L6
mirror "Mirror1" about plane through (0, 0, 0) normal (1, 0, 0) of "Extrude3"
sketch "Sketch6" plane through (0, 0, -22.5) normal (0, 0, -1) x (-1, 0, 0)
  line L0 (-22.5, 0) -> (22.5, 0)
  line L1 (22.5, 0) -> (22.5, 45)
  line L2 (22.5, 45) -> (-22.5, 45)
  line L3 (-22.5, 45) -> (-22.5, 0)
  line L4 (22.5, 27.25) -> (-22.5, 27.25)
  line L5 (-22.5, 27.25) -> (-22.5, 17.75)
  line L6 (-22.5, 17.75) -> (22.5, 17.75)
  line L7 (22.5, 17.75) -> (22.5, 27.25)
  line L8 (22.5, 27.25) -> (-22.5, 17.75) construction
  line L9 (-22.5, 27.25) -> (22.5, 17.75) construction
  line L10 (0, 0) -> (0, 6.5) construction
  line L11 (12.5, 27.25) -> (-12.5, 27.25)
  line L12 (-12.5, 27.25) -> (-12.5, 17.75)
  line L13 (-12.5, 17.75) -> (12.5, 17.75)
  line L14 (12.5, 17.75) -> (12.5, 27.25)
  line L15 (12.5, 27.25) -> (-12.5, 17.75) construction
  line L16 (-12.5, 27.25) -> (12.5, 17.75) construction
  point P0 (0, 22.5)
  point P1 (0, 22.5)
  dimension "d31" = 9.5
  dimension "d32" = 22.5
  dimension "d35" = 25
  constraint perpendicular L4 L5
  constraint parallel L4 L6
  constraint parallel L5 L7
  constraint horizontal L4
  constraint coincident L8 P1
  constraint coincident L9 P1
  constraint coincident L10.start origin
  constraint vertical L10
  constraint coincident P1 L10
  constraint coincident L1.end L7
  constraint perpendicular L11 L12
  constraint parallel L11 L13
  constraint parallel L12 L14
  constraint horizontal L11
  constraint coincident L4 L11.start
  constraint coincident L15 P1
  constraint coincident L16 P1
  constraint coincident P1 P0
  measures "d31" distance of L4 L6
  measures "d32" distance of L10.start P1
  measures "d35" distance of L12 L14
extrude "Extrude7" add sketch "Sketch6" along normal blind 3 contours L3 L4 L5 L6 L12 | L1 L4 L6 L7 L14
sketch "Sketch4" plane through (0, 0, -18.5) normal (0, 0, 1) x (1, 0, 0)
  line L0 (18.5, 45) -> (-18.5, 45)
  line L1 (-18.5, 45) -> (-18.5, 4)
  line L2 (-18.5, 4) -> (18.5, 4)
  line L3 (22.5, 45) -> (-22.5, 45)
  line L4 (-22.5, 0) -> (22.5, 0)
  line L5 (0, 0) -> (0, 20.1593) construction
  circle A0 centre (0, 22.5) radius 3.25
  dimension "d29" = 6.5
  dimension "d30" = 22.5
  constraint coincident L5.start origin
  constraint perpendicular L2 L5
  constraint coincident L5 A0.centre
  measures "d29" diameter of A0
  measures "d30" distance of L5.start A0.centre
extrude "Extrude5" cut sketch "Sketch4" against normal through all
sketch "Sketch5" plane through (0, 0, 0) normal (0, -1, 0) x (1, 0, 0)
  line L0 (22.5, -22.5) -> (22.5, 22.5)
  line L1 (-22.5, 22.5) -> (-22.5, -22.5)
  line L2 (-22.5, -22.5) -> (22.5, -22.5)
  line L3 (-22.5, -22.5) -> (22.5, -22.5)
  circle A0 centre (0, 0) radius 6.4
  dimension "d28" = 12.8
  constraint coincident A0.centre origin
  measures "d28" diameter of A0
extrude "Extrude6" cut sketch "Sketch5" against normal blind 4
equation "d30 = ( 45 / 2 ) * 1 mm"
equation "d32 = ( 45 / 2 ) * 1 mm"

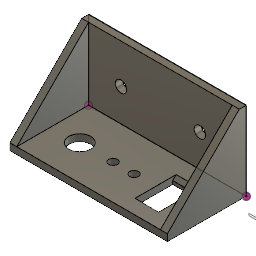
design "Switch Bracket"
Autodesk Fusion 360 part; units mm, degrees
sketch "Sketch1" plane through (0, 0, 0) normal (0, 1, 0) x (1, 0, 0)
  line L0 (45, 22.5) -> (-45, 22.5)
  line L1 (-45, 22.5) -> (-45, -22.5)
  line L2 (-45, -22.5) -> (45, -22.5)
  line L3 (45, -22.5) -> (45, 22.5)
  line L4 (45, 22.5) -> (-45, -22.5) construction
  line L5 (-45, 22.5) -> (45, -22.5) construction
  dimension "d1" = 45
  dimension "d2" = 90
  constraint perpendicular L0 L1
  constraint parallel L0 L2
  constraint parallel L1 L3
  constraint horizontal L0
  constraint coincident L4 origin
  constraint coincident L5 origin
  measures "d1" distance of L0.start L2.end L0.end
  measures "d2" distance of L0.start L0.end
extrude "Extrude1" add sketch "Sketch1" along normal blind 4
sketch "Sketch2" plane through (0, 0, -22.5) normal (0, 0, -1) x (-1, 0, 0)
  line L0 (45, 0) -> (-45, 0)
  line L1 (-45, 0) -> (-45, 45)
  line L2 (-45, 45) -> (45, 45)
  line L3 (45, 45) -> (45, 0)
  point P0 (-45, 0)
  point P1 (45, 0)
  dimension "d12" = 45
  constraint horizontal L0
  constraint vertical L1
  constraint horizontal L2
  constraint vertical L3
  constraint coincident L0 P0
  constraint coincident L1 P0
  constraint coincident L3 P1
  measures "d12" distance of P0 L1.end
extrude "Extrude4" add sketch "Sketch2" against normal blind 4
sketch "Sketch3" plane through (-45, 0, 0) normal (-1, 0, 0) x (0, 0, 1)
  line L0 (-22.5, 0) -> (22.5, 0)
  line L1 (22.5, 0) -> (22.5, 4)
  line L2 (22.5, 4) -> (-18.5, 4)
  line L3 (-22.5, 45) -> (-22.5, 0)
  line L4 (-18.5, 45) -> (-18.5, 4)
  line L5 (22.5, 4) -> (-18.5, 45)
  line L6 (-18.5, 4) -> (-18.5, 45)
  line L7 (-18.5, 45) -> (-22.5, 45)
  constraint coincident L2.end L4.end
  constraint coincident L1.end L2.start
  constraint coincident L4.start L5.end
extrude "Extrude3" add sketch "Sketch3" against normal blind 4 contours L2 L4 L5 L6
mirror "Mirror1" about plane through (0, 0, 0) normal (1, 0, 0) of "Extrude3"
sketch "Sketch4" plane through (0, 0, -18.5) normal (0, 0, 1) x (1, 0, 0)
  line L0 (41, 4) -> (41, 45)
  line L1 (41, 45) -> (-41, 45)
  line L2 (-41, 45) -> (-41, 4)
  line L3 (-41, 4) -> (41, 4)
  circle A0 centre (-22.5, 22.5) radius 3.25
  line L4 (-22.5, 22.5) -> (-16, 22.5) construction
  line L5 (45, 45) -> (-45, 45)
  line L6 (-45, 0) -> (45, 0)
  line L7 (0, 0) -> (0, 21) construction
  circle A1 centre (22.5, 22.5) radius 3.25
  dimension "d15" = 6.5
  dimension "d16" = 45
  constraint coincident A0.centre L4.start
  constraint horizontal L4
  constraint symmetric L4 L5 L6
  constraint coincident L7.start origin
  constraint perpendicular L3 L7
  constraint symmetric A0 L7 A1
  measures "d15" diameter of A0
  measures "d16" distance of A0.centre A1.centre
extrude "Extrude5" cut sketch "Sketch4" against normal through all contours A0 | A1
sketch "Sketch5" plane through (0, 0, 0) normal (0, -1, 0) x (1, 0, 0)
  line L0 (45, -22.5) -> (45, 22.5)
  line L1 (45, 22.5) -> (-45, 22.5)
  line L2 (-45, 22.5) -> (-45, -22.5)
  line L3 (-45, -22.5) -> (45, -22.5)
  circle A0 centre (-25, 2.5) radius 6.25
  line L4 (18.25, 12.25) -> (31.75, 12.25)
  line L5 (31.75, 12.25) -> (31.75, -7.25)
  line L6 (31.75, -7.25) -> (18.25, -7.25)
  line L7 (18.25, -7.25) -> (18.25, 12.25)
  line L8 (-25, 2.5) -> (31.5002, 2.5) construction
  line L9 (-45, -22.5) -> (45, -22.5)
  line L10 (25, -13) -> (25, 19) construction
  line L11 (-25, 2.5) -> (-25, -11) construction
  line L12 (0, 0) -> (0, -11) construction
  circle A1 centre (-6, 2.5) radius 2.5
  circle A2 centre (6, 2.5) radius 2.5
  dimension "d18" = 12.5
  dimension "d19" = 19.5
  dimension "d20" = 13.5
  dimension "d21" = 25
  dimension "d22" = 50
  dimension "d26" = 5
  dimension "d27" = 12
  constraint horizontal L4
  constraint vertical L5
  constraint horizontal L6
  constraint vertical L7
  constraint coincident A0.centre L8.start
  constraint horizontal L8
  constraint symmetric L4 L6 L8
  constraint perpendicular L4 L10
  constraint perpendicular L8 L11
  constraint coincident L12.start origin
  constraint vertical L12
  constraint coincident L8 A1.centre
  constraint symmetric L12 A1 A2
  measures "d18" diameter of A0
  measures "d19" distance of L4 L6
  measures "d20" distance of L4.start L4.end
  measures "d21" distance of L8 L9
  measures "d22" distance of A0.centre L10
  measures "d26" diameter of A1
  measures "d27" distance of A1.centre A2.centre
extrude "Extrude6" cut sketch "Sketch5" against normal blind 4 contours A0 | L4 L5 L6 L7 | A1 | A2
chamfer "Chamfer1" distance 2 angle 45 2 edges at (25, 4, -7.25) (25, 4, 12.25)
